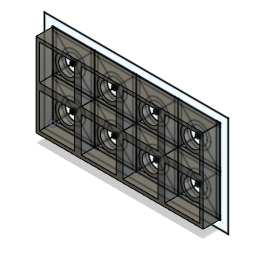
clear_led_array_panel (Autodesk Fusion 360 design; units mm, degrees)
Autodesk Fusion 360 part; units mm, degrees
note: some values were not read from the file. Set by a fixed rule: which sketch regions a step uses.
sketch "Sketch1" plane through (0, 0, 0) normal (0, 0, 1) x (1, 0, 0)
  line L0 (0, 0) -> (50, 0)
  line L1 (50, 0) -> (50, 25)
  line L2 (50, 25) -> (0, 25)
  line L3 (0, 25) -> (0, 0)
  line L4 (-2.5, -2.5) -> (52.5, -2.5)
  line L5 (52.5, -2.5) -> (52.5, 27.5)
  line L6 (52.5, 27.5) -> (-2.5, 27.5)
  line L7 (-2.5, 27.5) -> (-2.5, -2.5)
  line L8 (0, 25) -> (12.5, 25)
  line L9 (12.5, 25) -> (12.5, 12.5)
  line L10 (12.5, 12.5) -> (0, 12.5)
  line L11 (0, 12.5) -> (0, 25)
  line L12 (12.5, 12.5) -> (0, 12.5)
  line L13 (0, 12.5) -> (0, 0)
  line L14 (0, 0) -> (12.5, 0)
  line L15 (12.5, 0) -> (12.5, 12.5)
  line L16 (12.5, 12.5) -> (25, 12.5)
  line L17 (25, 12.5) -> (25, 25)
  line L18 (25, 25) -> (12.5, 25)
  line L19 (12.5, 25) -> (12.5, 12.5)
  line L20 (12.5, 12.5) -> (25, 12.5)
  line L21 (25, 12.5) -> (25, 0)
  line L22 (25, 0) -> (12.5, 0)
  line L23 (12.5, 0) -> (12.5, 12.5)
  line L24 (25, 12.5) -> (37.5, 12.5)
  line L25 (37.5, 12.5) -> (37.5, 25)
  line L26 (37.5, 25) -> (25, 25)
  line L27 (25, 25) -> (25, 12.5)
  line L28 (37.5, 12.5) -> (25, 12.5)
  line L29 (25, 12.5) -> (25, 0)
  line L30 (25, 0) -> (37.5, 0)
  line L31 (37.5, 0) -> (37.5, 12.5)
  line L32 (37.5, 12.5) -> (50, 12.5)
  line L33 (50, 12.5) -> (50, 0)
  line L34 (50, 0) -> (37.5, 0)
  line L35 (37.5, 0) -> (37.5, 12.5)
  line L36 (0, 25) -> (1, 25)
  line L37 (1, 25) -> (1, 0)
  line L38 (1, 0) -> (0, 0)
  line L39 (0, 0) -> (0, 25)
  line L40 (0, 25) -> (50, 25)
  line L41 (50, 25) -> (50, 24)
  line L42 (50, 24) -> (0, 24)
  line L43 (0, 24) -> (0, 25)
  line L44 (50, 0) -> (0, 0)
  line L45 (0, 0) -> (0, 1)
  line L46 (0, 1) -> (50, 1)
  line L47 (50, 1) -> (50, 0)
  line L48 (50, 25) -> (49, 25)
  line L49 (49, 25) -> (49, 0)
  line L50 (49, 0) -> (50, 0)
  line L51 (50, 0) -> (50, 25)
  line L52 (0, 12.5) -> (50, 12.5)
  line L53 (50, 12.5) -> (50, 11.5)
  line L54 (50, 11.5) -> (0, 11.5)
  line L55 (0, 11.5) -> (0, 12.5)
  line L56 (0, 12.5) -> (50, 12.5)
  line L57 (50, 12.5) -> (50, 13.5)
  line L58 (50, 13.5) -> (0, 13.5)
  line L59 (0, 13.5) -> (0, 12.5)
  line L60 (50, 25) -> (49, 25)
  line L61 (49, 25) -> (49, 0)
  line L62 (49, 0) -> (50, 0)
  line L63 (50, 0) -> (50, 25)
  line L64 (12.5, 0) -> (13.5, 0)
  line L65 (13.5, 0) -> (13.5, 25)
  line L66 (13.5, 25) -> (12.5, 25)
  line L67 (12.5, 25) -> (12.5, 0)
  line L68 (12.5, 25) -> (11.5, 25)
  line L69 (11.5, 25) -> (11.5, 0)
  line L70 (11.5, 0) -> (12.5, 0)
  line L71 (12.5, 0) -> (12.5, 25)
  line L72 (25, 25) -> (26, 25)
  line L73 (26, 25) -> (26, 0)
  line L74 (26, 0) -> (25, 0)
  line L75 (25, 0) -> (25, 25)
  line L76 (25, 25) -> (24, 25)
  line L77 (24, 25) -> (24, 0)
  line L78 (24, 0) -> (25, 0)
  line L79 (25, 0) -> (25, 25)
  line L80 (37.5, 25) -> (38.5, 25)
  line L81 (38.5, 25) -> (38.5, 0)
  line L82 (38.5, 0) -> (37.5, 0)
  line L83 (37.5, 0) -> (37.5, 25)
  line L84 (37.5, 25) -> (36.5, 25)
  line L85 (36.5, 25) -> (36.5, 0)
  line L86 (36.5, 0) -> (37.5, 0)
  line L87 (37.5, 0) -> (37.5, 25)
  line L88 (1, 24) -> (11.5, 13.5)
  line L89 (1, 13.5) -> (11.5, 24)
  line L90 (1, 11.5) -> (11.5, 1)
  line L91 (1, 1) -> (11.5, 11.5)
  line L92 (13.5, 24) -> (24, 13.5)
  line L93 (13.5, 13.5) -> (24, 24)
  line L94 (13.5, 11.5) -> (24, 1)
  line L95 (13.5, 1) -> (24, 11.5)
  line L96 (26, 11.5) -> (36.5, 1)
  line L97 (26, 1) -> (26, 1.4048)
  line L98 (36.5, 11.5) -> (26, 1)
  line L99 (36.5, 24) -> (26, 13.5)
  line L100 (26, 24) -> (36.5, 13.5)
  line L101 (38.5, 24) -> (49, 13.5)
  line L102 (38.5, 13.5) -> (49, 24)
  line L103 (38.5, 11.5) -> (49, 1)
  line L104 (38.5, 1) -> (49, 11.5)
  circle A0 centre (6.25, 18.75) radius 2.5
  circle A1 centre (18.75, 18.75) radius 2.5
  circle A2 centre (31.25, 18.75) radius 2.5
  circle A3 centre (43.75, 18.75) radius 2.5
  circle A4 centre (43.75, 6.25) radius 2.5
  circle A5 centre (31.25, 6.25) radius 2.5
  circle A6 centre (18.75, 6.25) radius 2.5
  circle A7 centre (6.25, 6.25) radius 2.5
  circle A8 centre (18.75, 6.25) radius 3.5
  circle A9 centre (31.25, 6.25) radius 3.5
  circle A10 centre (31.25, 18.75) radius 3.5
  circle A11 centre (18.75, 18.75) radius 3.5
  circle A12 centre (6.25, 18.75) radius 3.5
  circle A13 centre (43.75, 18.75) radius 3.5
  circle A14 centre (6.25, 6.25) radius 3.5
  circle A15 centre (43.75, 6.25) radius 3.5
  dimension "d1" = 50
  dimension "d2" = 25
  dimension "d3" = 2.5
  dimension "d4" = 12.5
  dimension "d5" = 12.5
  dimension "d6" = 12.5
  dimension "d7" = 12.5
  dimension "d8" = 12.5
  dimension "d9" = 12.5
  dimension "d10" = 12.5
  dimension "d11" = 12.5
  dimension "d12" = 12.5
  dimension "d13" = 12.5
  dimension "d14" = 12.5
  dimension "d15" = 1
  dimension "d16" = 1
  dimension "d17" = 1
  dimension "d18" = 1
  dimension "d19" = 25
  dimension "d20" = 50
  dimension "d21" = 1
  dimension "d22" = 50
  dimension "d23" = 1
  dimension "d24" = 1
  dimension "d25" = 1
  dimension "d26" = 25
  dimension "d27" = 1
  dimension "d28" = 1
  dimension "d29" = 1
  dimension "d30" = 1
  dimension "d31" = 5
  dimension "d32" = 5
  dimension "d33" = 5
  dimension "d34" = 5
  dimension "d35" = 5
  dimension "d36" = 5
  dimension "d37" = 5
  dimension "d38" = 5
  dimension "d39" = 1
  dimension "d40" = 1
  dimension "d41" = 1
  dimension "d42" = 1
  dimension "d43" = 1
  dimension "d44" = 1
  dimension "d51" = 1
  dimension "d52" = 1
  constraint horizontal L0
  constraint vertical L1
  constraint horizontal L2
  constraint vertical L3
  constraint coincident L0.start L3.end
  constraint horizontal L8
  constraint vertical L9
  constraint horizontal L10
  constraint vertical L11
  constraint horizontal L12
  constraint vertical L13
  constraint horizontal L14
  constraint vertical L15
  constraint horizontal L16
  constraint vertical L17
  constraint horizontal L18
  constraint vertical L19
  constraint horizontal L20
  constraint vertical L21
  constraint horizontal L22
  constraint vertical L23
  constraint horizontal L24
  constraint vertical L25
  constraint horizontal L26
  constraint vertical L27
  constraint horizontal L28
  constraint vertical L29
  constraint horizontal L30
  constraint vertical L31
  constraint horizontal L32
  constraint vertical L33
  constraint horizontal L34
  constraint vertical L35
  constraint horizontal L36
  constraint vertical L37
  constraint horizontal L38
  constraint vertical L39
  constraint horizontal L40
  constraint vertical L41
  constraint horizontal L42
  constraint vertical L43
  constraint horizontal L44
  constraint vertical L45
  constraint horizontal L46
  constraint vertical L47
  constraint horizontal L48
  constraint vertical L49
  constraint horizontal L50
  constraint vertical L51
  constraint horizontal L52
  constraint vertical L53
  constraint horizontal L54
  constraint vertical L55
  constraint horizontal L56
  constraint vertical L57
  constraint horizontal L58
  constraint vertical L59
  constraint horizontal L60
  constraint vertical L61
  constraint horizontal L62
  constraint vertical L63
  constraint horizontal L64
  constraint vertical L65
  constraint horizontal L66
  constraint vertical L67
  constraint horizontal L68
  constraint vertical L69
  constraint horizontal L70
  constraint vertical L71
  constraint horizontal L72
  constraint vertical L73
  constraint horizontal L74
  constraint vertical L75
  constraint horizontal L76
  constraint vertical L77
  constraint horizontal L78
  constraint vertical L79
  constraint horizontal L80
  constraint vertical L81
  constraint horizontal L82
  constraint vertical L83
  constraint horizontal L84
  constraint vertical L85
  constraint horizontal L86
  constraint vertical L87
  constraint coincident L37 L88.start
  constraint coincident L42 L88.start
  constraint coincident L69 L88.end
  constraint coincident L58 L88.end
  constraint coincident L58 L89.start
  constraint coincident L37 L89.start
  constraint coincident L69 L89.end
  constraint coincident L42 L89.end
  constraint coincident L37 L90.start
  constraint coincident L54 L90.start
  constraint coincident L69 L90.end
  constraint coincident L46 L90.end
  constraint coincident L37 L91.start
  constraint coincident L46 L91.start
  constraint coincident L69 L91.end
  constraint coincident L54 L91.end
  constraint perpendicular L90 L91
  constraint coincident L65 L92.start
  constraint coincident L42 L92.start
  constraint coincident L77 L92.end
  constraint coincident L58 L92.end
  constraint coincident L65 L93.start
  constraint coincident L58 L93.start
  constraint coincident L77 L93.end
  constraint coincident L42 L93.end
  constraint coincident L65 L94.start
  constraint coincident L54 L94.start
  constraint coincident L77 L94.end
  constraint coincident L46 L94.end
  constraint coincident L65 L95.start
  constraint coincident L46 L95.start
  constraint coincident L77 L95.end
  constraint coincident L54 L95.end
  constraint coincident L73 L96.start
  constraint coincident L54 L96.start
  constraint coincident L85 L96.end
  constraint coincident L46 L96.end
  constraint coincident L73 L97.start
  constraint coincident L46 L97.start
  constraint coincident L73 L97.end
  constraint coincident L85 L98.start
  constraint coincident L54 L98.start
  constraint coincident L85 L99.start
  constraint coincident L42 L99.start
  constraint coincident L73 L99.end
  constraint coincident L58 L99.end
  constraint coincident L73 L100.start
  constraint coincident L42 L100.start
  constraint coincident L85 L100.end
  constraint coincident L58 L100.end
  constraint coincident L81 L101.start
  constraint coincident L42 L101.start
  constraint coincident L49 L101.end
  constraint coincident L58 L101.end
  constraint coincident L81 L102.start
  constraint coincident L58 L102.start
  constraint coincident L49 L102.end
  constraint coincident L42 L102.end
  constraint perpendicular L101 L102
  constraint coincident L81 L103.start
  constraint coincident L54 L103.start
  constraint coincident L61 L103.end
  constraint coincident L46 L103.end
  constraint coincident L46 L104.start
  constraint coincident L81 L104.start
  constraint coincident L61 L104.end
  constraint coincident L54 L104.end
  constraint midpoint L88 A0.centre
  constraint midpoint L92 A1.centre
  constraint midpoint L99 A2.centre
  constraint midpoint L101 A3.centre
  constraint midpoint L103 A4.centre
  constraint midpoint L98 A5.centre
  constraint midpoint L94 A6.centre
  constraint midpoint L90 A7.centre
  measures "d1" distance of L0.start L0.end
  measures "d2" distance of L0.start L2.end
  measures "d4" distance of L2.end L8.end
  measures "d5" distance of L2.end L10.end
  measures "d6" distance of L9.end L16.end
  measures "d7" distance of L9.end L8.end
  measures "d8" distance of L9.end L16.end
  measures "d9" distance of L9.end L14.end
  measures "d10" distance of L16.end L24.end
  measures "d11" distance of L16.end L17.end
  measures "d12" distance of L24.end L16.end
  measures "d13" distance of L24.end L30.end
  measures "d14" distance of L24.end L32.end
  measures "d15" distance of L2.end L36.end
  measures "d16" distance of L2.end L42.end
  measures "d17" distance of L0.end L46.end
  measures "d18" distance of L1.end L48.end
  measures "d19" distance of L1.end L0.end
  measures "d20" distance of L10.end L32.end
  measures "d21" distance of L10.end L54.end
  measures "d22" distance of L10.end L32.end
  measures "d23" distance of L10.end L58.end
  measures "d24" distance of L14.end L64.end
  measures "d25" distance of L8.end L68.end
  measures "d26" distance of L8.end L14.end
  measures "d27" distance of L17.end L72.end
  measures "d28" distance of L17.end L76.end
  measures "d29" distance of L25.end L80.end
  measures "d30" distance of L25.end L84.end
  measures "d31" diameter of A0
  measures "d32" diameter of A1
  measures "d33" diameter of A2
  measures "d34" diameter of A3
  measures "d35" diameter of A4
  measures "d36" diameter of A5
  measures "d37" diameter of A6
  measures "d38" diameter of A7
extrude "Extrude2" add sketch "Sketch1" along normal blind 5 contours L0 L3 L13 L14 L37 L38 L39 L44 L45 L46 | L0 L14 L37 L44 L46 L69 | L3 L13 L37 L39 L46 L54 | L0 L14 L15 L23 L44 L46 L67 L69 L70 L71 | L3 L10 L12 L13 L37 L39 L52 L54 L55 L56 | L0 L15 L22 L23 L44 L46 L64 L65 L67 L71 | L15 L23 L46 L54 L67 L69 L71 | L10 L12 L37 L52 L54 L56 L69 | L3 L10 L11 L12 L37 L39 L52 L56 L58 L59 | L0 L22 L44 L46 L65 L77 | L15 L23 L46 L54 L65 L67 L71 | L10 L12 L15 L23 L52 L54 L56 L67 L69 L71 | L10 L12 L37 L52 L56 L58 L69 | L3 L11 L37 L39 L42 L58 | L0 L21 L22 L29 L44 L46 L75 L77 L78 L79 | L15 L16 L20 L23 L52 L54 L56 L65 L67 L71 | L9 L10 L12 L19 L52 L56 L58 L67 L69 L71 | L2 L3 L8 L11 L36 L37 L39 L40 L42 L43 | L0 L21 L29 L30 L44 L46 L73 L74 L75 L79 | L21 L29 L46 L54 L75 L77 L79 | L16 L20 L52 L54 L56 L65 L77 | L9 L16 L19 L20 L52 L56 L58 L65 L67 L71 | L9 L19 L42 L58 L67 L69 L71 | L2 L8 L37 L40 L42 L69 | L0 L30 L44 L46 L73 L85 | L21 L29 L46 L54 L73 L75 L79 L97 | L16 L20 L21 L29 L52 L54 L56 L75 L77 L79 | L16 L20 L52 L56 L58 L65 L77 | L9 L19 L42 L58 L65 L67 L71 | L2 L8 L9 L19 L40 L42 L67 L68 L69 L71 | L0 L30 L31 L35 L44 L46 L83 L85 L86 L87 | L21 L24 L28 L29 L52 L54 L56 L73 L75 L79 | L16 L17 L20 L27 L52 L56 L58 L75 L77 L79 | L2 L9 L18 L19 L40 L42 L65 L66 L67 L71 | L0 L31 L34 L35 L44 L46 L81 L82 L83 L87 | L31 L35 L46 L54 L83 L85 L87 | L17 L24 L27 L28 L52 L56 L58 L73 L75 L79 | L24 L28 L52 L54 L56 L73 L85 | L17 L27 L42 L58 L75 L77 L79 | L2 L18 L40 L42 L65 L77 | L0 L34 L44 L46 L49 L61 L81 | L31 L35 L46 L54 L81 L83 L87 | L24 L28 L31 L35 L52 L54 L56 L83 L85 L87 | L17 L27 L42 L58 L73 L75 L79 | L24 L28 L52 L56 L58 L73 L85 | L2 L17 L18 L27 L40 L42 L75 L76 L77 L79 | L0 L1 L33 L34 L44 L46 L47 L49 L50 L51 L61 L62 L63 | L31 L32 L35 L52 L54 L56 L81 L83 L87 | L24 L25 L28 L52 L56 L58 L83 L85 L87 | L2 L17 L26 L27 L40 L42 L72 L73 L75 L79 | L1 L33 L46 L49 L51 L54 L61 L63 | L32 L49 L52 L54 L56 L61 L81 | L25 L32 L52 L56 L58 L81 L83 L87 | L25 L42 L58 L83 L85 L87 | L2 L26 L40 L42 L73 L85 | L1 L32 L33 L49 L51 L52 L53 L54 L56 L61 L63 | L32 L49 L52 L56 L58 L61 L81 | L25 L42 L58 L81 L83 L87 | L2 L25 L26 L40 L42 L83 L84 L85 L87 | L1 L32 L49 L51 L52 L56 L57 L58 L61 L63 | L2 L25 L40 L42 L80 L81 L83 L87 | L1 L42 L49 L51 L58 L61 L63 | L2 L40 L42 L49 L61 L81 | L1 L2 L40 L41 L42 L48 L49 L51 L60 L61 L63 makes body 1
extrude "Extrude1" add sketch "Sketch1" along normal blind 2 separate body contours L90 L91 A7 A14 | L90 L91 A7 A14 | L90 L91 A7 A14 | L90 L91 A7 A14 | L94 L95 A6 A8 | L94 L95 A6 A8 | L88 L89 A0 A12 | L88 L89 A0 A12 | L94 L95 A6 A8 | L94 L95 A6 A8 | L88 L89 A0 A12 | L88 L89 A0 A12 | L96 L98 A5 A9 | L96 L98 A5 A9 | L92 L93 A1 A11 | L92 L93 A1 A11 | L96 L98 A5 A9 | L96 L98 A5 A9 | L92 L93 A1 A11 | L92 L93 A1 A11 | L103 L104 A4 A15 | L103 L104 A4 A15 | L99 L100 A2 A10 | L99 L100 A2 A10 | L103 L104 A4 A15 | L103 L104 A4 A15 | L99 L100 A2 A10 | L99 L100 A2 A10 | L101 L102 A3 A13 | L101 L102 A3 A13 | L101 L102 A3 A13 | L101 L102 A3 A13 makes body 2 at (9.7326, 19.0985, 1.3333) makes body 3 at (34.7326, 6.5985, 1.3333) makes body 4 at (22.2326, 19.0985, 1.3333) makes body 5 at (34.7326, 19.0985, 1.3333) makes body 6 at (22.2326, 6.5985, 1.3333) makes body 7 at (47.2326, 6.5985, 1.3333) makes body 8 at (47.2326, 19.0985, 1.3333) makes body 9 at (9.7326, 6.5985, 1.3333)
extrude "Extrude3" add sketch "Sketch1" along normal blind 1 contours L37 L90 L91 A14 | L69 L90 L91 A14 | L90 L91 A7 A14 | L90 L91 A7 A14 | L65 L94 L95 A8 | L37 L88 L89 A12 | L77 L94 L95 A8 | L69 L88 L89 A12 | L73 L96 L97 L98 A9 | L65 L92 L93 A11 | L85 L96 L98 A9 | L77 L92 L93 A11 | L81 L103 L104 A15 | L73 L99 L100 A10 | L49 L61 L103 L104 A15 | L103 L104 A4 A15 | L85 L99 L100 A10 | L103 L104 A4 A15 | L81 L101 L102 A13 | L49 L61 L101 L102 A13 picked at (3.824, 4.2265) picked at (9.3996, 5.9889) picked at (41.0607, 4.5923) picked at (46.0898, 4.1256) bodies 7 1 3 4 5 6 8 9 2
